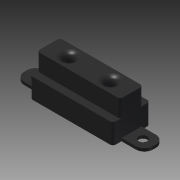
# Autodesk Inventor part: PSDセンサ
Saved by Autodesk Inventor 2015 (Build 190159000, 159)
## iProperties
Created: 2015-05-10
Part Number: PSDセンサ
Material: アセタール樹脂、黒
Document SubType Name: Modeling
Designer: kenta
Density: 0.762685 g/cm^3
Appearance: オキシダイズド
Mass: 3 g
Surface Area: 21.8266 cm^2
Volume: 3.93347 cm^3
Author: kenta
Autodesk Inventor part; units mm, degrees
ref_plane "YZ Plane" through (0, 0, 0) normal (1, 0, 0) x (0, 1, 0)
ref_plane "XZ Plane" through (0, 0, 0) normal (0, 1, 0) x (-1, 0, 0)
ref_plane "XY Plane" through (0, 0, 0) normal (0, 0, 1) x (1, 0, 0)
sketch "スケッチ1" plane through (0, 0, 0) normal (0, 0, 1) x (1, 0, 0)
  line L0 (-22.5, 6.5) -> (22.5, 6.5)
  line L1 (22.5, 6.5) -> (22.5, -6.5)
  line L2 (22.5, -6.5) -> (-22.5, -6.5)
  line L3 (-22.5, -6.5) -> (-22.5, 6.5)
  line L4 (-22.5, 6.5) -> (22.5, -6.5) construction
  line L5 (22.5, 6.5) -> (-22.5, -6.5) construction
  point P0 (0, 0)
  dimension "d0" = 45
  dimension "d1" = 13
  constraints: 12 end point, 2 midpoint, 2 parallel, 1 horizontal, 1 perpendicular
  measures "d0" distance of L1.end L2.end
  measures "d1" distance of L0.end L1.end
extrude "押し出し1" add sketch "スケッチ1" along normal blind 1
sketch "スケッチ2" plane through (0, 0, 1) normal (0, 0, 1) x (1, 0, 0)
  line L0 (-14.5, 6.5) -> (14.5, 6.5)
  line L1 (14.5, 6.5) -> (14.5, -6.5)
  line L2 (14.5, -6.5) -> (-14.5, -6.5)
  line L3 (-14.5, -6.5) -> (-14.5, 6.5)
  line L4 (-14.5, 6.5) -> (14.5, -6.5) construction
  line L5 (14.5, 6.5) -> (-14.5, -6.5) construction
  point P0 (0, 0)
  dimension "d4" = 29
  dimension "d5" = 13
  constraints: 12 end point, 2 midpoint, 2 parallel, 1 horizontal, 1 perpendicular
  measures "d4" distance of L1.end L2.end
  measures "d5" distance of L0.end L1.end
extrude "押し出し2" add sketch "スケッチ2" along normal blind 6
sketch "スケッチ4" plane through (0, 0, 7) normal (0, 0, 1) x (1, 0, 0)
  line L0 (-14.5, 4) -> (14.5, 4)
  line L1 (14.5, 4) -> (14.5, -4)
  line L2 (14.5, -4) -> (-14.5, -4)
  line L3 (-14.5, -4) -> (-14.5, 4)
  line L4 (-14.5, 4) -> (14.5, -4) construction
  line L5 (14.5, 4) -> (-14.5, -4) construction
  point P0 (0, 0)
  dimension "d8" = 29
  dimension "d9" = 8
  constraints: 12 end point, 2 midpoint, 2 parallel, 1 horizontal, 1 perpendicular
  measures "d8" distance of L1.end L2.end
  measures "d9" distance of L0.end L1.end
extrude "押し出し3" add sketch "スケッチ4" along normal blind 6
sketch "スケッチ5" plane through (0, 0, 1) normal (0, 0, 1) x (1, 0, 0)
  point P0 (0, 0)
sketch "スケッチ6" plane through (0, 0, 1) normal (0, 0, 1) x (1, 0, 0)
  line L0 (22.5, 6.5) -> (14.5, 6.5)
  line L1 (14.5, 6.5) -> (14.5, 3.5)
  line L2 (14.5, 3.5) -> (22.5, 3.5)
  line L3 (22.5, 3.5) -> (22.5, 6.5)
  line L4 (22.5, -6.5) -> (14.5, -6.5)
  line L5 (14.5, -6.5) -> (14.5, -3.5)
  line L6 (14.5, -3.5) -> (22.5, -3.5)
  line L7 (22.5, -3.5) -> (22.5, -6.5)
  line L8 (-22.5, 6.5) -> (-14.5, 6.5)
  line L9 (-14.5, 6.5) -> (-14.5, 3.5)
  line L10 (-14.5, 3.5) -> (-22.5, 3.5)
  line L11 (-22.5, 3.5) -> (-22.5, 6.5)
  line L12 (-22.5, -6.5) -> (-14.5, -6.5)
  line L13 (-14.5, -6.5) -> (-14.5, -3.5)
  line L14 (-14.5, -3.5) -> (-22.5, -3.5)
  line L15 (-22.5, -3.5) -> (-22.5, -6.5)
  point P0 (0, 0)
  dimension "d12" = 8
  dimension "d13" = 3
  dimension "d14" = 8
  dimension "d15" = 3
  dimension "d16" = 8
  dimension "d17" = 3
  dimension "d18" = 8
  dimension "d19" = 3
  constraints: 32 end point, 8 parallel, 4 horizontal, 4 perpendicular, 2 point on line
  measures "d12" distance of L2.end L1.end
  measures "d13" distance of L1.end L0.end
  measures "d14" distance of L5.end L6.end
  measures "d15" distance of L4.end L5.end
  measures "d16" distance of L9.end L10.end
  measures "d17" distance of L8.end L9.end
  measures "d18" distance of L14.end L13.end
  measures "d19" distance of L13.end L12.end
extrude "押し出し4" cut sketch "スケッチ6" against normal blind 6
fillet "フィレット1" radius 3 4 edges at (22.5, 3.5, 0.5) (22.5, -3.5, 0.5) (-22.5, 3.5, 0.5) (-22.5, -3.5, 0.5)
sketch "スケッチ7" plane through (0, 0, 13) normal (0, 0, 1) x (1, 0, 0)
  point P0 (0, 0)
  point P1 (7.25, 0)
  point P2 (-7.25, 0)
  point P3 (-18.5, 0)
  point P4 (18.5, 0)
hole "穴1" at (7.25, 0, 13) at (-7.25, 0, 13) at (-18.5, 0, 13) at (18.5, 0, 13) direction (0, 0, -1) diameter 3 end through all
fillet "フィレット2" radius 2 2 edges at (-7.25, 1.5, 13) (7.25, 1.5, 13)
sketch "スケッチ8" plane through (0, 0, 0) normal (0, 0, -1) x (-1, 0, 0)
  line L0 (12.5, -3.5) -> (-12.5, -3.5)
  line L1 (-12.5, -3.5) -> (-12.5, 3.5)
  line L2 (-12.5, 3.5) -> (12.5, 3.5)
  line L3 (12.5, 3.5) -> (12.5, -3.5)
  line L4 (12.5, -3.5) -> (-12.5, 3.5) construction
  line L5 (-12.5, -3.5) -> (12.5, 3.5) construction
  point P0 (0, 0)
  dimension "d31" = 7
  dimension "d32" = 25
  constraints: 12 end point, 2 midpoint, 2 parallel, 1 horizontal, 1 perpendicular
  measures "d31" distance of L2.end L0.start
  measures "d32" distance of L1.end L2.end
extrude "押し出し5" cut sketch "スケッチ8" against normal blind 2
sketch "スケッチ9" plane through (0, 0, 2) normal (0, 0, -1) x (-1, 0, 0)
  line L0 (12.5, -3.5) -> (-12.5, -3.5)
  line L1 (-12.5, -3.5) -> (-12.5, 3.5)
  line L2 (-12.5, 3.5) -> (12.5, 3.5)
  line L3 (12.5, 3.5) -> (12.5, -3.5)
  line L4 (12.5, -3.5) -> (-12.5, 3.5) construction
  line L5 (-12.5, -3.5) -> (12.5, 3.5) construction
  point P0 (0, 0)
  dimension "d35" = 25
  dimension "d36" = 7
  constraints: 12 end point, 2 midpoint, 2 parallel, 1 horizontal, 1 perpendicular
  measures "d35" distance of L1.end L2.end
  measures "d36" distance of L0.end L1.end
extrude "押し出し6" add sketch "スケッチ9" along normal blind 2
fillet "フィレット3" radius 1 8 edges at (14.5, 4, 10) (14.5, 6.5, 3.5) (14.5, -4, 10) (14.5, -6.5, 3.5) (-14.5, 6.5, 3.5) (-14.5, 4, 10) (-14.5, -4, 10) (-14.5, -6.5, 3.5)
